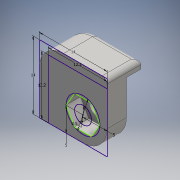
# Autodesk Inventor part: RxBoardMountFootWithNut
Saved by Autodesk Inventor 2016 (Build 200138000, 138)
## iProperties
Created: 2026-04-05
Part Number: RxBoardMountFootWithNut
Material: Generic
Document SubType Name: Modeling
Designer: Steve
Density: 1 g/cm^3
Appearance: Default
Author: Steve
Autodesk Inventor part; units mm, degrees
ref_plane "YZ Plane" through (0, 0, 0) normal (1, 0, 0) x (0, 1, 0)
ref_plane "XZ Plane" through (0, 0, 0) normal (0, 1, 0) x (-1, 0, 0)
ref_plane "XY Plane" through (0, 0, 0) normal (0, 0, 1) x (1, 0, 0)
sketch "Sketch1" plane through (0, 0, 0) normal (0, 1, 0) x (-1, 0, 0)
  line L0 (0, 0) -> (14, 0)
  line L1 (14, 0) -> (14, 14)
  line L2 (14, 14) -> (0, 14)
  line L3 (0, 14) -> (0, 0)
  circle A0 centre (5, 5) radius 1.75
  line L4 (0, 0) -> (12.2, 0)
  line L5 (12.2, 0) -> (12.2, 12.2)
  line L6 (12.2, 12.2) -> (0, 12.2)
  line L7 (0, 12.2) -> (0, 0)
  circle A1 centre (5, 5) radius 3.5
  line L8 (1.5, 5) -> (3.25, 8.0311)
  line L9 (3.25, 8.0311) -> (6.75, 8.0311)
  line L10 (6.75, 8.0311) -> (8.5, 5)
  line L11 (8.5, 5) -> (6.75, 1.9689)
  line L12 (6.75, 1.9689) -> (3.25, 1.9689)
  line L13 (3.25, 1.9689) -> (1.5, 5)
  dimension "d19" = 7
  dimension "d0" = 14
  dimension "d1" = 14
  dimension "d2" = 3.5
  dimension "d3" = 5
  dimension "d4" = 5
  dimension "d5" = 12.2
  dimension "d6" = 12.2
  constraints: 28 end point, 4 parallel, 2 coincident, 2 horizontal, 2 perpendicular, 1 centre point, 1 horizontal alignment, 15 other
  measures "d0" distance of L2.end L1.end
  measures "d1" distance of L1.end L0.end
  measures "d2" diameter of A0
  measures "d3" distance from line of L0 A0.centre
  measures "d4" distance from line of L3 A0.centre
  measures "d5" distance of L6.end L5.end
  measures "d6" distance of L5.end L4.end
extrude "Extrusion3" add sketch "Sketch1" along normal blind 4 contours L3 L6 L5 L0 | L10 A1 | L11 L12 L13 L8 L9 L10 | A1 L11 | L9 A1 | A1 L12 | L8 A1 | A1 L13
extrude "Extrusion4" add sketch "Sketch1" along normal blind 7 contours L5 L6 L3 L2 L1 L0
fillet "Fillet3" radius 5 3 edges at (0, 2, 0) (-12.2, 5.5, 12.2) (-14, 3.5, 14)
fillet "Fillet4" radius 1 5 edges at (-12.5355, 7, 12.5355) (-4.5, 7, 14) (-14, 7, 4.5) (-14, 3.5, 0) (0, 3.5, 14)
extrude "Extrusion5" cut sketch "Sketch1" along normal blind 3 contours L11 L12 L13 L8 L9 L10
body "Solid2"
